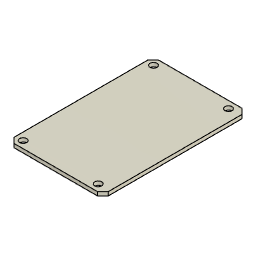
Side Panel - Blank Template (Autodesk Fusion 360 design; units mm, degrees)
Autodesk Fusion 360 part; units mm, degrees
ref_plane "WorkPlane2" through (0, 0, 2.999) normal (0, 0, 1) x (1, 0, 0)
sketch "Sketch4" plane through (0, 0, 2.999) normal (0, 0, 1) x (1, 0, 0)
  line L0 (92.5002, -5.0854) -> (92.4954, -5.0854)
  line L1 (89.5002, -5.0854) -> (44.5002, -5.0854) construction
  line L2 (44.5002, -5.0854) -> (41.5002, -8.0854) construction
  line L3 (41.5002, -8.0854) -> (41.5002, -80.0854) construction
  line L4 (41.5002, -80.0854) -> (44.5002, -83.0854) construction
  line L5 (44.5002, -83.0854) -> (89.5002, -83.0854) construction
  line L6 (92.5002, -80.0854) -> (92.5002, -8.0854) construction
  line L7 (86.0002, -79.0854) -> (86.0002, -83.0854) construction
  line L8 (86.0002, -79.0854) -> (92.5002, -79.0854) construction
  line L9 (86.0002, -79.0854) -> (45.705, -79.088) construction
  line L10 (45.7002, -79.0828) -> (41.5002, -79.0831) construction
  line L11 (45.7002, -9.088) -> (45.7002, -5.0854) construction
  line L12 (45.7002, -9.088) -> (45.705, -79.088) construction
  line L13 (45.6956, -9.088) -> (85.9956, -9.0854) construction
  line L14 (85.9956, -9.0854) -> (92.5002, -9.0854) construction
  line L15 (85.9956, -9.0854) -> (85.9956, -5.0854) construction
  line L16 (85.9956, -79.0854) -> (85.9931, -9.0854) construction
  line L17 (92.5002, -80.0854) -> (89.5002, -83.0854) construction
  line L18 (92.5002, -8.0854) -> (89.5002, -5.0854) construction
  line L19 (44.583, -82.8854) -> (89.4174, -82.8854)
  line L20 (92.3002, -80.0026) -> (89.4174, -82.8854)
  line L21 (92.3002, -80.0026) -> (92.3002, -8.1683)
  line L22 (92.3002, -8.1683) -> (89.4174, -5.2854)
  line L23 (89.4174, -5.2854) -> (44.583, -5.2854)
  line L24 (44.583, -5.2854) -> (41.7002, -8.1683)
  line L25 (41.7002, -8.1683) -> (41.7002, -80.0026)
  line L26 (41.7002, -80.0026) -> (44.583, -82.8854)
  circle A0 centre (85.9956, -9.0854) radius 1.9
  circle A1 centre (45.7002, -9.088) radius 1.9
  circle A2 centre (85.9956, -79.0854) radius 1.9
  circle A3 centre (45.7002, -79.0828) radius 1.9
  line L27 (92.5002, -44.0854) -> (41.5002, -44.0854) construction
  point P0 (92.5002, -83.0854)
  point P1 (92.5002, -5.0854)
  dimension "d34" = 6.5
  dimension "d35" = 4
  dimension "d36" = 4.2
  dimension "d37" = 40.2952
  dimension "d38" = 4
  dimension "d39" = 3
  dimension "d40" = 3
  dimension "d43" = 78
  dimension "d44" = 3
  dimension "d45" = 3
  dimension "d46" = 3
  dimension "d47" = 3
  dimension "d48" = 3
  dimension "d49" = 3
  dimension "d50" = -0.2
  dimension "d53" = 3.8
  dimension "d54" = 3.8
  dimension "d55" = 3.8
  dimension "d56" = 3.8
  dimension "d57" = 51
  constraint coincident L5 L7.end
  constraint perpendicular L5 L7
  constraint coincident L6 L8.end
  constraint perpendicular L6 L8
  constraint coincident L3 L10.end
  constraint coincident L1 L11.end
  constraint perpendicular L1 L11
  constraint perpendicular L10 L12
  constraint coincident L6 L14.end
  constraint perpendicular L6 L14
  constraint coincident L1 L15.end
  constraint perpendicular L1 L15
  constraint horizontal L1
  constraint vertical L6
  constraint horizontal L5
  constraint vertical L3
  constraint coincident P0 L6
  constraint coincident P0 L5
  constraint coincident L6 P1
  constraint coincident L1 P1
  constraint coincident L0.start L6
  constraint coincident L0.end L1
  constraint coincident L13.end L14.start
  constraint coincident L11.start L12.start
  constraint coincident L16.start A2.centre
  constraint coincident L10.start A3.centre
  constraint midpoint L6 L27.start
  constraint midpoint L3 L27.end
  constraint symmetric A1 A3 L27
  constraint symmetric A0 A2 L27
  measures "d34" horizontal distance of L7.start L8.end
  measures "d35" vertical distance of L7.start L7.end
  measures "d36" horizontal distance of L10.start L10.end
  measures "d37" horizontal distance of L7.start L9.end
  measures "d38" vertical distance of L13.end L15.end
  measures "d39" horizontal distance of L1.end L2.end
  measures "d40" vertical distance of L1.end L2.end
  measures "d43" distance of L1 L5
  measures "d44" horizontal distance of L3.end L4.end
  measures "d45" vertical distance of L3.end L4.end
  measures "d46" distance of P0 L6.start
  measures "d47" distance of P0 L5.end
  measures "d48" distance of L6.end P1
  measures "d49" distance of L1.start P1
  measures "d53" diameter of A0
  measures "d54" diameter of A1
  measures "d55" diameter of A2
  measures "d56" diameter of A3
  measures "d57" distance of L3 L6
extrude "Extrude11" add sketch "Sketch4" against normal blind 2
equation "d39 = d40"
equation "d40 = d44"
equation "d45 = d44"
equation "d46 = d44"
equation "d47 = d46"
equation "d48 = d44"
equation "d49 = d48"
equation "d53 = d55"
equation "d54 = d55"
equation "d56 = d55"
